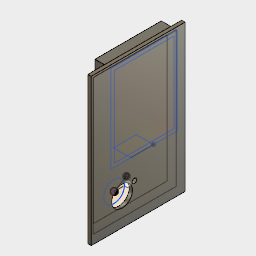
WeMOS D1 + sensor space (Autodesk Fusion 360 design; units mm, degrees)
Autodesk Fusion 360 part; units mm, degrees
sketch "Sketch1" plane through (0, 0, 0) normal (0, 0, 1) x (1, 0, 0) in component "D1 holder"
sketch "Sketch2" plane through (0, 0, 0) normal (1, 0, 0) x (0, 0, -1) in component "D1 holder"
  line L0 (-20.5, 32) -> (20.5, 32)
  line L1 (20.5, 32) -> (20.5, -32)
  line L2 (20.5, -32) -> (-20.5, -32)
  line L3 (-20.5, -32) -> (-20.5, 32)
  line L4 (-20.5, 32) -> (20.5, -32) construction
  line L5 (20.5, 32) -> (-20.5, -32) construction
  dimension "d27" = 41
  dimension "d28" = 64
  measures "d27" distance of L1.end L2.end
  measures "d28" distance of L0.end L1.end
extrude "Extrude1" add sketch "Sketch2" along normal blind 1.5 makes body 1 in component "D1 holder"
sketch "Sketch3" plane through (1.5, 0, 0) normal (1, 0, 0) x (0, 0, -1) in component "D1 holder"
  line L0 (-20.5, -32) -> (20.5, -32)
  line L1 (20.5, -32) -> (20.5, 32)
  line L2 (20.5, 32) -> (-20.5, 32)
  line L3 (-20.5, 32) -> (-20.5, -32)
  line L4 (-18.1, 29.6) -> (-18.1, -29.6)
  line L5 (-18.1, -29.6) -> (18.1, -29.6)
  line L6 (18.1, -29.6) -> (18.1, 29.6)
  line L7 (18.1, 29.6) -> (-18.1, 29.6)
  dimension "d31" = 2.4
extrude "Extrude2" add sketch "Sketch3" along normal blind 2 contours L4 L5 L6 L7 bodies 1 in component "D1 holder"
sketch "Sketch4" plane through (3.5, 0, 0) normal (1, 0, 0) x (0, 0, -1) in component "D1 holder"
  line L0 (18.1, 29.6) -> (-18.1, 29.6)
  line L1 (-18.1, 29.6) -> (-18.1, -29.6)
  line L2 (-18.1, -29.6) -> (18.1, -29.6)
  line L3 (18.1, -29.6) -> (18.1, 29.6)
  line L4 (-16.1, 27.6) -> (-16.1, -27.6)
  line L5 (-16.1, -27.6) -> (16.1, -27.6)
  line L6 (16.1, -27.6) -> (16.1, 27.6)
  line L7 (16.1, 27.6) -> (-16.1, 27.6)
  dimension "d34" = 2
extrude "Extrude3" cut sketch "Sketch4" against normal blind 2 contours L4 L5 L6 L7 bodies 1 in component "D1 holder"
sketch "Sketch8" plane through (1.5, 0, 0) normal (1, 0, 0) x (0, 0, -1) in component "D1 holder"
  line L0 (18.5846, -29.167) -> (-10.4154, -29.167)
  line L1 (-10.4154, -29.167) -> (-10.4154, 8.833)
  line L2 (-10.4154, 8.833) -> (18.5846, 8.833)
  line L3 (18.5846, 8.833) -> (18.5846, -29.167)
  line L4 (17.0846, -27.667) -> (-8.9154, -27.667)
  line L5 (-8.9154, -27.667) -> (-8.9154, 7.333)
  line L6 (-8.9154, 7.333) -> (17.0846, 7.333)
  line L7 (17.0846, 7.333) -> (17.0846, -27.667)
  dimension "d39" = 29
  dimension "d40" = 38
  dimension "d41" = 1.5
  measures "d39" distance of L0.start L0.end
  measures "d40" distance of L0.start L2.end
extrude "Extrude4" add sketch "Sketch8" along normal blind 7 separate body makes body 2 in component "D1 holder"
sketch "Sketch9" plane through (0, 8.833, 0) normal (0, 1, 0) x (-1, 0, 0) in component "D1 holder"
  line L0 (-1.5, -18.5846) -> (-1.5, 10.4154)
  line L1 (-1.5, 10.4154) -> (-8.5, 10.4154)
  line L2 (-8.5, 10.4154) -> (-8.5, -18.5846)
  line L3 (-8.5, -18.5846) -> (-1.5, -18.5846)
  line L4 (-1.5, -8.142) -> (-8.9091, -8.142)
  line L5 (-8.9091, -8.142) -> (-8.9091, 1.858)
  line L6 (-8.9091, 1.858) -> (-1.5, 1.858)
  line L7 (-1.5, 1.858) -> (-1.5, -8.142)
  dimension "d44" = 10
  measures "d44" distance of L4.start L6.end
extrude "Extrude5" cut sketch "Sketch9" against normal blind 1.5 contours L0 L2 L4 L6 L7 bodies 2 in component "D1 holder"
sketch "sensor hole" plane through (3.5, 0, 0) normal (1, 0, 0) x (0, 0, -1) in component "D1 holder"
  circle A0 centre (-7.0063, 20.0021) radius 4.5
  dimension "d47" = 9
  measures "d47" diameter of A0
extrude "Extrude6" cut sketch "sensor hole" against normal blind 26 bodies 1 in component "D1 holder"
sketch "screw hole" plane through (3.5, 0, 0) normal (1, 0, 0) x (0, 0, -1) in component "D1 holder"
  line L0 (-7.0063, 20.0021) -> (-1.6369, 16.9021)
  line L1 (-7.0063, 20.0021) -> (-1.0063, 20.0021) construction
  circle A0 centre (-1.6369, 16.9021) radius 1
  point P0 (-7.0063, 20.0021)
  dimension "d130" = 30
  dimension "d131" = 6.2
  dimension "d132" = 2
  measures "d130" angle of L0 L1
  measures "d131" distance of P0 L0.end
  measures "d132" diameter of A0
extrude "Extrude7" cut sketch "screw hole" against normal blind 4 bodies 1 in component "D1 holder"
component "D1 holder" placed x (-1, 0, 0) y (0, -1, 0) z (0, 0, 1) at (0, 0, 0)
